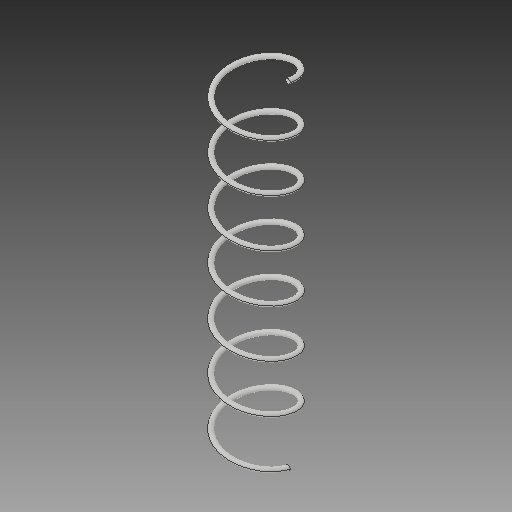
# Autodesk Inventor part: vis infini_CPY
Saved by Autodesk Inventor 2019 (Build 230136000, 136)
## iProperties
Created: 2018-12-30
Part Number: vis infini_CPY
Material: Générique
Document SubType Name: Modeling
Designer: pouey
Density: 1 g/cm^3
Appearance: Par défaut
Author: pouey
Autodesk Inventor part; units mm, degrees
ref_plane "YZ Plane" through (0, 0, 0) normal (1, 0, 0) x (0, 1, 0)
ref_plane "XZ Plane" through (0, 0, 0) normal (0, 1, 0) x (-1, 0, 0)
ref_plane "XY Plane" through (0, 0, 0) normal (0, 0, 1) x (1, 0, 0)
sketch "Esquisse2" plane through (0, 0, 0) normal (0, 0, 1) x (1, 0, 0)
  line L0 (0, 0) -> (0, 20)
  line L1 (0, 0) -> (20, 0)
  circle A0 centre (20, 0) radius 1.5
  dimension "d0" = 20
  dimension "d1" = 20
  dimension "d2" = 3
  constraints: 4 end point, 1 centre point, 1 coincident, 1 horizontal, 1 vertical
  measures "d0" distance of L0.start L0.end
  measures "d1" distance of L0.start L1.end
  measures "d2" diameter of A0
coil "Hélicoïde1" sketch "Esquisse2" operation add axis through (0, 0, 0) along (0, -1, 0) pitch 30 turns 7 hand left
